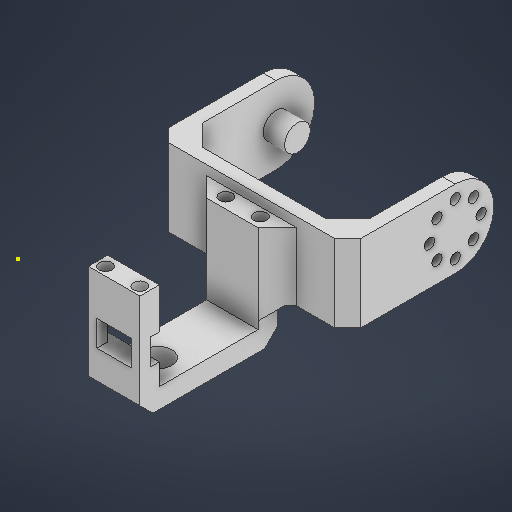
# Autodesk Inventor part: Arm1
Saved by Autodesk Inventor 2026 (Build 300175050, 175E)
## iProperties
Created: 2026-07-07
Part Number: Arm1
Material: 一般
Document SubType Name: Modeling
Designer: hanaj
Density: 1 g/cm^3
Appearance: 既定
Author: hanaj
Autodesk Inventor part; units mm, degrees
ref_plane "YZ Plane" through (0, 0, 0) normal (1, 0, 0) x (0, 1, 0)
ref_plane "XZ Plane" through (0, 0, 0) normal (0, 1, 0) x (-1, 0, 0)
ref_plane "XY Plane" through (0, 0, 0) normal (0, 0, 1) x (1, 0, 0)
sketch "スケッチ1" plane through (0, 0, 0) normal (1, 0, 0) x (0, 1, 0)
  circle A0 centre (0, 0) radius 9
  line L0 (9, 0) -> (-9, 0)
  line L1 (-9, 0) -> (-9, 25)
  line L2 (-9, 25) -> (9, 25)
  line L3 (9, 25) -> (9, 0)
  dimension "d0" = 18
  dimension "d1" = 25
  dimension "d2" = 18
  constraints: 8 end point, 2 parallel, 2 point on circle, 1 centre point, 1 coincident, 1 horizontal, 1 perpendicular
  measures "d0" diameter of A0
  measures "d1" distance of L0.end L1.end
  measures "d2" distance of L1.end L2.end
extrude "押し出し1" add sketch "スケッチ1" along normal blind 3
sketch "スケッチ2" plane through (3, 0, 0) normal (1, 0, 0) x (0, 0, -1)
  line L0 (-25, 9) -> (-25, -9) projected
  line L1 (-25, -9) -> (-22, -9)
  line L2 (-22, -9) -> (-22, 9)
  line L3 (-22, 9) -> (-25, 9)
  line L4 (-25, 9) -> (-25, -9)
  line L5 (0, 9) -> (-25, 9) projected
  point P0 (0, 0)
  point P1 (-25, 9)
  dimension "d5" = 3
  constraints: 8 end point, 2 parallel, 1 collinear, 1 horizontal, 1 perpendicular
  measures "d5" distance between parallel lines of L2 L0
extrude "押し出し2" add sketch "スケッチ2" along normal blind 38.7
sketch "スケッチ3" plane through (41.7, 0, 0) normal (1, 0, 0) x (0, 0, -1)
  line L0 (-22, 9) -> (-22, -9) projected
  line L1 (-22, -9) -> (0, -9) projected
  arc A0 (0, -9) -> (0, 9) centre (0, 0) ccw projected
  line L2 (0, 9) -> (-22, 9) projected
  line L3 (-22, -9) -> (-22, 9) projected
  line L4 (-22, 9) -> (-25, 9) projected
  line L5 (-25, 9) -> (-25, -9) projected
  line L6 (-25, -9) -> (-22, -9) projected
extrude "押し出し3" add sketch "スケッチ3" along normal blind 3
sketch "スケッチ4" plane through (0, -9, 25) normal (0, 0, 1) x (1, 0, 0)
  line L0 (28.35, 22.75) -> (16.35, 22.75)
  line L1 (16.35, 22.75) -> (16.35, -4.75)
  line L2 (16.35, -4.75) -> (28.35, -4.75)
  line L3 (28.35, -4.75) -> (28.35, 22.75)
  line L4 (28.35, 22.75) -> (16.35, -4.75) construction
  line L5 (16.35, 22.75) -> (28.35, -4.75) construction
  line L6 (44.7, 18) -> (44.7, 0) projected
  line L7 (0, 0) -> (44.7, 0) projected
  line L8 (28.35, 15.75) -> (16.35, 15.75)
  point P0 (0, 9)
  point P1 (22.35, 9)
  dimension "d10" = 12
  dimension "d11" = 27.5
  dimension "d12" = 22.35
  dimension "d13" = 9
  dimension "d16" = 7
  constraints: 14 end point, 2 midpoint, 2 parallel, 2 perpendicular, 2 point on line, 1 horizontal
  measures "d10" distance of L2.end L1.end
  measures "d11" distance of L1.end L0.end
  measures "d12" distance from line of L6 point (22.35, 9)
  measures "d13" distance from line of L7 point (22.35, 9)
  measures "d16" distance between parallel lines of L8 L0
extrude "押し出し4" add sketch "スケッチ4" along normal blind 4.5 contours L3 L7 L1 L8 | L3 L2 L1 L7
sketch "スケッチ5" plane through (0, -9, 25) normal (0, 0, -1) x (-1, 0, 0)
  line L0 (-28.35, -4.75) -> (-28.35, 0) projected
  line L1 (-28.35, -4.75) -> (-16.35, -4.75)
  line L2 (-16.35, -4.75) -> (-16.35, -10.35)
  line L3 (-16.35, -10.35) -> (-28.35, -10.35)
  line L4 (-28.35, -10.35) -> (-28.35, -4.75)
  line L5 (-16.35, 15.75) -> (-16.35, -4.75) projected
  point P0 (0, 9)
  dimension "d17" = 5.6
  constraints: 8 end point, 2 parallel, 1 collinear, 1 horizontal, 1 perpendicular
  measures "d17" distance between parallel lines of L3 L1
extrude "押し出し5" add sketch "スケッチ5" against normal blind 32
sketch "スケッチ6" plane through (16.35, -13.75, 29.5) normal (0, 1, 0) x (1, 0, 0)
  line L0 (0, 0) -> (0, -27.5) projected
  line L1 (12, -27.5) -> (0, -27.5)
  line L2 (0, -27.5) -> (0, -23)
  line L3 (0, -23) -> (12, -23)
  line L4 (12, -23) -> (12, -27.5)
  line L5 (12, -27.5) -> (0, -27.5) projected
  line L6 (12, 0) -> (12, -27.5) projected
  point P0 (-16.35, 29.5)
  point P1 (6, -23)
  point P2 (0, -27.5)
  dimension "d20" = 4.5
  constraints: 8 end point, 2 collinear, 2 parallel, 1 horizontal, 1 midpoint, 1 perpendicular, 1 point on line
  measures "d20" distance from line of point (6, -23) L1
extrude "押し出し6" add sketch "スケッチ6" along normal blind 20.5
sketch "スケッチ7" plane through (44.7, 0, 0) normal (1, 0, 0) x (0, 0, -1)
  circle A0 centre (0, 0) radius 6 construction
  line L0 (7.5318, 0) -> (-7.5318, 0) construction
  point P0 (-6, 0)
  point P1 (-4.2426, -4.2426)
  point P2 (0, -6)
  point P3 (4.2426, -4.2426)
  point P4 (6, 0)
  point P5 (4.2426, 4.2426)
  point P6 (0, 6)
  point P7 (-4.2426, 4.2426)
  dimension "d23" = 12
  dimension "d26" = 360
  constraints: 2 end point, 1 coincident, 1 horizontal, 1 horizontal alignment, 1 midpoint, 1 point on line, 11 other
hole "穴1" at (44.7, 0, 6) at (44.7, -4.2426, 4.2426) at (44.7, -6, 0) at (44.7, -4.2426, -4.2426) at (44.7, 0, -6) at (44.7, 4.2426, -4.2426) at (44.7, 6, 0) at (44.7, 4.2426, 4.2426) direction (-1, 0, 0) diameter 2.4 depth 6.3 clearance for "Countersunk Flat Head Screw ISO 2009/7046" size "M2" standard "ISO"
sketch "スケッチ8" plane through (16.35, -19.35, 25) normal (0, -1, 0) x (1, 0, 0)
  line L0 (0, 32) -> (12, 32) construction
  line L1 (6, 32) -> (6, 0) construction
  line L2 (0, 0) -> (12, 0) construction
  point P0 (-16.35, -25)
  point P1 (6, 21.79)
  dimension "d35" = 10.21
  constraints: 2 end point, 2 midpoint, 1 point on line
  measures "d35" distance from line of point (6, 21.79) L0
hole "穴2" at (22.35, -19.35, 46.79) direction (0, 1, 0) diameter 6.4 depth 6.3
sketch "スケッチ9" plane through (16.35, -19.35, 25) normal (0, -1, 0) x (1, 0, 0)
  circle A0 centre (6, 21.79) radius 3.2 projected
  line L0 (12, 0) -> (0, 0) projected
  line L1 (12, 0) -> (12, 32) projected
  line L2 (0, 32) -> (12, 32) projected
  line L3 (0, 0) -> (0, 32) projected
  point P0 (-16.35, -25)
extrude "押し出し7" cut sketch "スケッチ9" against normal blind 1
sketch "スケッチ10" plane through (3, 0, 0) normal (1, 0, 0) x (0, 0, -1)
  circle A0 centre (0, 0) radius 3
  dimension "d45" = 6
  constraints: 1 centre point, 1 coincident
  measures "d45" diameter of A0
extrude "押し出し8" add sketch "スケッチ10" along normal blind 5
sketch "スケッチ11" plane through (16.35, 6.75, 29.5) normal (0, 1, 0) x (1, 0, 0)
  circle A0 centre (6, -17.29) radius 3.2 projected
  line L0 (6, -51.8359) -> (6, 17.2559)
  line L1 (37.0866, -11.5) -> (-25.0866, -11.5)
  line L2 (0, -27.5) -> (12, -27.5) projected
  line L3 (-16.35, 4.5) -> (28.35, 4.5) projected
  point P0 (-16.35, 29.5)
  point P1 (6, -11.5)
  point P2 (10, 2.5)
  point P3 (2, 2.5)
  point P4 (10, -25.5)
  point P5 (2, -25.5)
  dimension "d48" = 16
  dimension "d49" = 8
  dimension "d50" = 2
  constraints: 4 end point, 3 symmetric about line, 2 midpoint, 1 horizontal, 1 point on line, 1 vertical
  measures "d48" distance between parallel lines of L1 L2
  measures "d49" diameter of point (10, 2.5) L0
  measures "d50" distance from line of L3 point (10, 2.5)
hole "穴3" at (26.35, 6.75, 27) at (18.35, 6.75, 27) at (26.35, 6.75, 55) at (18.35, 6.75, 55) direction (0, -1, 0) diameter 3 depth 3
chamfer "面取り1" distance 5 angle 45 2 edges at (41.7, 0, 22) (3, 0, 22)
chamfer "面取り2" distance 3 angle 45 2 edges at (22.35, -18.35, 57) (22.35, -18.35, 25)
chamfer "面取り3" distance 4.5 angle 45 2 edges at (16.35, -1.125, 25) (28.35, -1.125, 25)
chamfer "面取り4" distance 3 angle 45 3 edges at (22.35, -9, 25) (16.35, -9, 27.2499) (28.35, -9, 27.2499)
chamfer "面取り5" distance 3 angle 45 2 edges at (0, 0, 25) (44.7, 0, 25)
sketch "スケッチ12" plane through (0, -9, 57) normal (0, 0, 1) x (1, 0, 0)
  point P0 (0, 9)
sketch "スケッチ13" plane through (0, -9, 57) normal (0, 0, 1) x (1, 0, 0)
  line L0 (26.35, 6.25) -> (18.35, 6.25)
  line L1 (18.35, 6.25) -> (18.35, 0.25)
  line L2 (18.35, 0.25) -> (26.35, 0.25)
  line L3 (26.35, 0.25) -> (26.35, 6.25)
  line L4 (26.35, 6.25) -> (18.35, 0.25) construction
  line L5 (18.35, 6.25) -> (26.35, 0.25) construction
  line L6 (16.35, -4.75) -> (28.35, -4.75) projected
  line L7 (28.35, -6.35) -> (28.35, 15.75) projected
  point P0 (0, 9)
  point P1 (22.35, 3.25)
  dimension "d73" = 6
  dimension "d74" = 8
  dimension "d75" = 5
  dimension "d76" = 6
  constraints: 12 end point, 2 midpoint, 2 parallel, 1 horizontal, 1 perpendicular
  measures "d73" distance of L2.end L0.start
  measures "d74" distance of L1.end L2.end
  measures "d75" distance between parallel lines of L6 L2
  measures "d76" distance from line of point (22.35, 3.25) L7
extrude "押し出し9" cut sketch "スケッチ13" against normal blind 10
sketch "スケッチ14" plane through (28.35, -13.75, 52.5) normal (1, 0, 0) x (0, 0, -1)
  line L0 (0, 11) -> (0, 5) projected
  line L1 (-4.5, 11) -> (0, 11) projected
  line L2 (-4.5, 5) -> (-4.5, 11) projected
  line L3 (-4.5, 5) -> (0, 5) projected
  line L4 (-2, 5) -> (-2, 11)
  point P0 (52.5, 13.75)
  dimension "d79" = 2
  constraints: 2 end point, 2 point on line, 1 perpendicular
  measures "d79" distance between parallel lines of L0 L4
extrude "押し出し10" cut sketch "スケッチ14" against normal through all contours L0 L3 L4 L1
